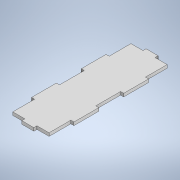
# Autodesk Inventor part: base
Saved by Autodesk Inventor 2020 (Build 240168000, 168)
## iProperties
Created: 2020-02-22
Part Number: base
Material: Generic
Document SubType Name: Modeling
Designer: udvarhelyi
Density: 1 g/cm^3
Appearance: Default
Author: udvarhelyi
Autodesk Inventor part; units mm, degrees
ref_plane "YZ Plane" through (0, 0, 0) normal (1, 0, 0) x (0, 1, 0)
ref_plane "XZ Plane" through (0, 0, 0) normal (0, 1, 0) x (-1, 0, 0)
ref_plane "XY Plane" through (0, 0, 0) normal (0, 0, 1) x (1, 0, 0)
sketch "Sketch1" plane through (0, 0, 0) normal (0, 1, 0) x (-1, 0, 0)
  line L0 (-2.5, -54) -> (-2.5, -54)
  line L1 (-2.5, -54) -> (2.5, -54)
  line L2 (2.5, -54) -> (2.5, -54)
  line L3 (-12.5, -54) -> (-12.5, -54)
  line L4 (-12.5, -54) -> (-7.5, -54)
  line L5 (-7.5, -54) -> (-7.5, -54)
  line L6 (12.5, -54) -> (12.5, -54)
  line L7 (12.5, -54) -> (7.5, -54)
  line L8 (7.5, -54) -> (7.5, -54)
  line L9 (7.5, 60) -> (7.5, 60)
  line L10 (7.5, 60) -> (12.5, 60)
  line L11 (12.5, 60) -> (12.5, 60)
  line L12 (-2.5, 60) -> (-2.5, 60)
  line L13 (-2.5, 60) -> (2.5, 60)
  line L14 (2.5, 60) -> (2.5, 60)
  line L15 (-12.5, 60) -> (-12.5, 60)
  line L16 (-12.5, 60) -> (-7.5, 60)
  line L17 (-7.5, 60) -> (-7.5, 60)
  line L18 (17.5, 60) -> (17.5, 60)
  line L19 (17.5, -54) -> (17.5, -54)
  line L20 (-17.5, 60) -> (-17.5, 60)
  line L21 (-17.5, -54) -> (-17.5, -54)
  line L22 (17.5, -54) -> (17.5, -54)
  line L23 (17.5, 60) -> (17.5, 60)
  line L24 (12.5, -54) -> (17.5, -54)
  line L25 (2.5, -54) -> (7.5, -54)
  line L26 (-17.5, -54) -> (-12.5, -54)
  line L27 (-7.5, -54) -> (-2.5, -54)
  line L28 (-17.5, 60) -> (-17.5, 60)
  line L29 (-17.5, -54) -> (-17.5, -54)
  line L30 (-12.5, 60) -> (-17.5, 60)
  line L31 (-2.5, 60) -> (-7.5, 60)
  line L32 (17.5, 60) -> (12.5, 60)
  line L33 (7.5, 60) -> (2.5, 60)
  line L34 (17.5, -33) -> (20.5, -33)
  line L35 (20.5, -33) -> (20.5, -9)
  line L36 (20.5, -9) -> (17.5, -9)
  line L37 (17.5, 39) -> (20.5, 39)
  line L38 (20.5, 39) -> (20.5, 15)
  line L39 (20.5, 15) -> (17.5, 15)
  line L40 (-17.5, 39) -> (-20.5, 39)
  line L41 (-20.5, 39) -> (-20.5, 15)
  line L42 (-20.5, 15) -> (-17.5, 15)
  line L43 (-17.5, -9) -> (-20.5, -9)
  line L44 (-20.5, -9) -> (-20.5, -33)
  line L45 (-20.5, -33) -> (-17.5, -33)
  line L46 (17.5, -33) -> (17.5, -54)
  line L47 (17.5, 60) -> (17.5, 39)
  line L48 (17.5, 15) -> (17.5, -9)
  line L49 (-17.5, 60) -> (-17.5, 39)
  line L50 (-17.5, 15) -> (-17.5, -9)
  line L51 (-17.5, -33) -> (-17.5, -54)
  line L52 (5.8333, 60) -> (-5.8333, 60)
  line L53 (-5.8333, 60) -> (-5.8333, 63)
  line L54 (-5.8333, 63) -> (5.8333, 63)
  line L55 (5.8333, 63) -> (5.8333, 60)
  line L56 (5.8333, -54) -> (-5.8333, -54)
  line L57 (-5.8333, -54) -> (-5.8333, -57)
  line L58 (-5.8333, -57) -> (5.8333, -57)
  line L59 (5.8333, -57) -> (5.8333, -54)
  point P0 (0, 0)
  point P1 (-17.5, 50)
  point P2 (-17.5, -44)
  point P3 (17.5, -44)
  point P4 (17.5, 50)
  point P5 (-5.8333, 60)
  dimension "d40" = 35
  dimension "d49" = 0
  dimension "d50" = 0
  dimension "d55" = 17.5
  dimension "d56" = 60
  dimension "d57" = 114
  dimension "d58" = 0
  dimension "d59" = 0
  dimension "d62" = 24
  dimension "d63" = 24
  dimension "d65" = 3
  dimension "d66" = 21
  dimension "d67" = 11.6667
  dimension "d68" = 11.6667
  dimension "d69" = 3
  dimension "d70" = 3
  constraints: 120 end point, 38 parallel, 22 collinear, 21 perpendicular, 20 point on line, 12 horizontal, 7 equal length, 1 other
  measures "d40" distance of L26.start L22.start
  measures "d49" distance of L19.start L19.end
  measures "d50" distance of L21.start L21.end
  measures "d55" distance from line of L28 point (0, 0)
  measures "d56" distance from line of point (0, 0) L31
  measures "d57" distance between parallel lines of L30 L26
  measures "d58" distance from line of L32 L18.end
  measures "d59" distance from line of L24 L19.start
  measures "d62" distance of L37.end L38.end
  measures "d63" distance of L39.end L36.end
  measures "d65" distance of L34.start L34.end
  measures "d66" distance of L18.end L37.start
  measures "d67" distance of L53.end L54.end
  measures "d68" distance between parallel lines of L49 L53
  measures "d69" distance of L54.end L52.start
  measures "d70" distance of L56.end L57.end
extrude "Extrusion1" add sketch "Sketch1" along normal blind 3
equation "\"d40\" = shelfH"
equation "\"d55\" = 0.5 * shelfH"
equation "\"d56\" = 0.5 * ht"
equation "\"d57\" = -2 * tt + ht"
equation "\"d62\" = 0.2 * ht + 2 * tol"
equation "\"d63\" = 0.2 * ht - 2 * tol"
equation "\"d65\" = tt"
equation "\"d66\" = 0.2 * ht - tt"
equation "\"d67\" = 0.333333 * shelfH + 2 * tol"
equation "\"d68\" = 0.333333 * shelfH - tol"
equation "\"d69\" = tt"
equation "\"d70\" = tt"
equation "\"d31\" = tt"
equation "\"d4\" = tt"
equation "\"tt\" = 3"
equation "\"tol\" = 0"
equation "\"tiroir\" = 1"
equation "\"nHoles\" = 4"
equation "\"shelfH\" = 35"
equation "\"d42\" = 0.5 * shelfH"
equation "\"d43\" = 0.5 * shelfH"
equation "\"ht\" = 120"
body "Solid1"
